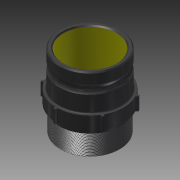
# Autodesk Inventor part: deliverance
Saved by Autodesk Inventor 2013 SP2 (Build 170200200, 200)
## iProperties
Created: 2013-09-06
Part Number: deliverance
Material: GFRP
Document SubType Name: Modeling
Designer: mrister
Density: 1.75 g/cm^3
Description: Cam Lock - 3" Male Adapter x Male Thr'd, (BANJO 300F)
Engineer: mrister
Mass: 751.241 g
Surface Area: 358.727 cm^2
Volume: 92.9754 cm^3
Author: mrister
Autodesk Inventor part; units mm, degrees
ref_plane "YZ Plane" through (0, 0, 0) normal (1, 0, 0) x (0, 1, 0)
ref_plane "XZ Plane" through (0, 0, 0) normal (0, 1, 0) x (-1, 0, 0)
ref_plane "XY Plane" through (0, 0, 0) normal (0, 0, 1) x (1, 0, 0)
sketch "Sketch1" plane through (0, 0, 0) normal (0, 0, 1) x (1, 0, 0)
  line L0 (-45.6406, 0) -> (-45.6406, 23.8125)
  arc A0 (-45.6406, 23.8125) -> (-45.6406, 36.5125) centre (-51.5087, 30.1625) ccw
  line L1 (-45.6406, 36.5125) -> (-45.6406, 52.3875)
  line L2 (-45.6406, 52.3875) -> (-38.989, 52.3875)
  line L3 (-38.989, 52.3875) -> (-38.989, 0)
  line L4 (-38.989, 0) -> (-45.6406, 0)
  line L5 (-38.989, 0) -> (0, 0) construction
  line L6 (-45.6406, 0) -> (-49.6094, 0)
  line L7 (-49.6094, 0) -> (-49.6094, -19.05)
  line L8 (-49.6094, -19.05) -> (-44.45, -19.05)
  line L9 (-44.45, -19.05) -> (-44.45, -57.15)
  line L10 (-44.45, -57.15) -> (-38.989, -57.15)
  line L11 (-38.989, -57.15) -> (-38.989, 0)
  line L12 (0, -79.0575) -> (0, 74.295) projected
  point P0 (-42.8625, 30.1625)
  dimension "d5" = 12.7
  dimension "d28" = 38.989
  dimension "d29" = 22.225
  dimension "d30" = 42.8625
  dimension "d31" = 45.6406
  dimension "d32" = 44.45
  dimension "d33" = 49.6094
  dimension "d34" = 109.5375
  dimension "d35" = 38.1
  dimension "d60" = 19.05
  constraints: 24 end point, 6 parallel, 3 collinear, 3 point on circle, 2 perpendicular, 1 centre point, 1 coincident, 1 horizontal, 1 vertical
  measures "d5" distance of L0.end L1.start
  measures "d28" distance from line of point (0, 0) L3
  measures "d29" distance from line of A0.centre L2
  measures "d30" horizontal distance of point (0, 0) point (-42.862, 30.162)
  measures "d31" distance from line of point (0, 0) L1
  measures "d32" distance from line of point (0, 0) L9
  measures "d33" distance from line of L5.end L7
  measures "d34" distance between parallel lines of L2 L10
  measures "d35" distance of L8.end L9.end
  measures "d60" distance of L6.end L7.end
revolve "Revolution1" add sketch "Sketch1" angle 360 about axis through (0, -10, 0) along (0, 1, 0)
sketch "Sketch4" plane through (0, 0, 0) normal (0, 1, 0) x (-1, 0, 0)
  line L0 (-1.5875, 52.759) -> (1.5875, 52.759)
  line L1 (1.5875, 52.759) -> (1.5875, 49.584)
  line L2 (1.5875, 49.584) -> (-1.5875, 49.584)
  line L3 (-1.5875, 49.584) -> (-1.5875, 52.759)
  line L4 (0, 49.584) -> (0, 0) construction
  circle A0 centre (0, 0) radius 49.6094 construction
  line L5 (-46.4844, 25.0047) -> (-44.8969, 27.7543)
  line L6 (-44.8969, 27.7543) -> (-42.1472, 26.1668)
  line L7 (-42.1472, 26.1668) -> (-43.7347, 23.4172)
  line L8 (-43.7347, 23.4172) -> (-46.4844, 25.0047)
  line L9 (-44.8969, -27.7543) -> (-46.4844, -25.0047)
  line L10 (-46.4844, -25.0047) -> (-43.7347, -23.4172)
  line L11 (-43.7347, -23.4172) -> (-42.1472, -26.1668)
  line L12 (-42.1472, -26.1668) -> (-44.8969, -27.7543)
  line L13 (1.5875, -52.759) -> (-1.5875, -52.759)
  line L14 (-1.5875, -52.759) -> (-1.5875, -49.584)
  line L15 (-1.5875, -49.584) -> (1.5875, -49.584)
  line L16 (1.5875, -49.584) -> (1.5875, -52.759)
  line L17 (46.4844, -25.0047) -> (44.8969, -27.7543)
  line L18 (44.8969, -27.7543) -> (42.1472, -26.1668)
  line L19 (42.1472, -26.1668) -> (43.7347, -23.4172)
  line L20 (43.7347, -23.4172) -> (46.4844, -25.0047)
  line L21 (44.8969, 27.7543) -> (46.4844, 25.0047)
  line L22 (46.4844, 25.0047) -> (43.7347, 23.4172)
  line L23 (43.7347, 23.4172) -> (42.1472, 26.1668)
  line L24 (42.1472, 26.1668) -> (44.8969, 27.7543)
  point P0 (-42.941, 24.792)
  point P1 (-42.941, -24.792)
  point P2 (0, -49.584)
  point P3 (42.941, -24.792)
  point P4 (42.941, 24.792)
  dimension "d36" = 3.175
  dimension "d38" = 3.175
  dimension "d41" = 360
  constraints: 50 end point, 2 parallel, 1 horizontal, 1 midpoint, 1 perpendicular, 1 vertical, 57 other
  measures "d36" distance of L0.start L0.end
  measures "d38" distance of L0.end L1.end
extrude "Extrusion3" add sketch "Sketch4" against normal blind 19.05
chamfer "Chamfer3" distance 1.5875 angle 45 4 edges at (45.6406, 52.3875, 0) (38.989, 52.3875, 0) (44.45, -57.15, 0) (38.989, -57.15, 0)
fillet "Fillet2" radius 1.5875 14 edges at (44.45, -19.05, 0) (45.6406, 0, 0) (43.7347, -9.525, 23.4172) (42.1472, -9.525, -26.1668) (1.5875, -9.525, -49.584) (43.7347, -9.525, -23.4172) (42.1472, -9.525, 26.1668) (1.5875, -9.525, 49.584) (-1.5875, -9.525, 49.584) (-42.1472, -9.525, 26.1668) (-43.7347, -9.525, -23.4172) (-43.7347, -9.525, 23.4172) (-42.1472, -9.525, -26.1668) (-1.5875, -9.525, -49.584)
sketch "Sketch5" plane through (0, 0, 0) normal (0, 0, 1) x (1, 0, 0)
  line L0 (-44.45, -55.5625) -> (-44.45, -20.6375) projected
  line L1 (-43.6562, -64.6353) -> (-44.45, -65.0322)
  line L2 (-44.45, -65.0322) -> (-44.45, -64.2384)
  line L3 (-43.6562, -64.6353) -> (-44.45, -64.6353) construction
  line L4 (-43.6562, -64.6353) -> (-44.45, -64.2384)
  point P0 (0, 0)
  dimension "d49" = 0.7937
  dimension "d51" = 0.7937
  constraints: 8 end point, 2 collinear, 1 horizontal, 1 midpoint
  measures "d49" distance of L1.end L2.end
  measures "d51" distance of L1.start L3.end
coil "Coil1" sketch "Sketch5" operation cut axis through (0, -10, 0) along (0, 1, 0) pitch 0.9525 turns 40 hand right
equation "\"d51\" = d49"
body "Solid1"
